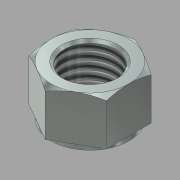
# Autodesk Inventor part: Hex Nut with Washer Face
Saved by Autodesk Inventor 2011 SP2 (Build 150309200, 309)
## iProperties
Created: 2014-10-30
Part Number: Hex Nut with Washer Face
Document SubType Name: Modeling
Designer: Greg Pavlik
Density: 1 g/cm^3
Author: Greg Pavlik
Autodesk Inventor part; units mm, degrees
ref_plane "YZ Plane" through (0, 0, 0) normal (1, 0, 0) x (0, 1, 0)
ref_plane "XZ Plane" through (0, 0, 0) normal (0, 1, 0) x (-1, 0, 0)
ref_plane "XY Plane" through (0, 0, 0) normal (0, 0, 1) x (1, 0, 0)
sketch "Sketch1" plane through (0, 0, 0) normal (0, 0, 1) x (1, 0, 0)
  line L0 (0, 2.5981) -> (2.25, 1.299)
  line L1 (2.25, 1.299) -> (2.25, -1.299)
  line L2 (2.25, -1.299) -> (0, -2.5981)
  line L3 (0, -2.5981) -> (-2.25, -1.299)
  line L4 (-2.25, -1.299) -> (-2.25, 1.299)
  line L5 (-2.25, 1.299) -> (0, 2.5981)
  circle A0 centre (0, 0) radius 1.5 construction
  dimension "Diameter" = 3
  dimension "Width_Across_Flats" = 4.5
  constraints: 12 end point, 2 coincident, 1 centre point, 1 vertical, 13 other
  measures "Diameter" diameter of A0
  measures "Width_Across_Flats" distance between parallel lines of L0 L3
extrude "Extrusion1" add sketch "Sketch1" along normal mid plane 2.625
sketch "Sketch2" plane through (0, 0, 0) normal (0, 1, 0) x (-1, 0, 0)
  line L0 (-2.25, 1.3125) -> (-2.25, -1.3125) construction
  line L1 (0, 0) -> (0, 4.375)
  line L2 (-2.25, 1.3125) -> (-3.75, 1.3125)
  line L3 (-3.75, 1.3125) -> (-3.75, 0.4465)
  line L4 (-3.75, 0.4465) -> (-2.25, 1.3125)
  dimension "Chamfer_Angle" = 30
  dimension "Chamfer_Size" = 1.5
  constraints: 8 end point, 2 perpendicular, 1 parallel
  measures "Chamfer_Angle" angle of L4 L2
  measures "Chamfer_Size" distance of L0.start L2.end
revolve "Revolution1" cut sketch "Sketch2" angle 360 about axis through (0, 0, 0) along (0, 0, 1)
sketch "Sketch3" plane through (0, 0, -1.3125) normal (0, 0, -1) x (-1, 0, 0)
  line L0 (2.25, -1.299) -> (0, -2.5981) construction
  circle A0 centre (0, 0) radius 2.25
  constraints: 1 centre point, 1 coincident, 1 tangent
extrude "Extrusion2" add sketch "Sketch3" along normal blind 0.25
hole "Hole1" at (0, 0, 1.3125) direction (0, 0, -1) diameter 3 end through all
thread "Thread1" size "M3x0.5" class "6H" standard "ANSI Metric M Profile" full length
chamfer "Chamfer1" distance 0.15 angle 45 2 edges at (0, 1.5, 1.3125) (0, 1.5, -1.5625)
equation "\"Width_Across_Flats\" = 1.5 * Diameter"
equation "\"Thickness\" = 0.875 * Diameter"
equation "\"Chamfer_Size\" = 0.5 * Diameter"
equation "\"Hole_Diameter\" = Diameter"
body "Solid1"
